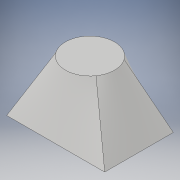
# Autodesk Inventor part: 410571040-4
Saved by Autodesk Inventor 2017 (Build 210142000, 142)
## iProperties
Part Number: 410571040-4
Material: 一般
Document SubType Name: Modeling
Designer: user
Density: 1 g/cm^3
Appearance: 預設
Author: user
Autodesk Inventor part; units mm, degrees
ref_plane "YZ Plane" through (0, 0, 0) normal (1, 0, 0) x (0, 1, 0)
ref_plane "XY Plane" through (0, 0, 0) normal (0, 0, 1) x (1, 0, 0)
sketch "草圖1" plane through (0, 0, 0) normal (0, 1, 0) x (-1, 0, 0)
  line L0 (0, 0) -> (-100, 0)
  line L1 (-100, 0) -> (-100, -70)
  line L2 (-100, -70) -> (0, -70)
  line L3 (0, -70) -> (0, 0)
  dimension "d0" = 100
  dimension "d1" = 70
  constraints: 8 end point, 3 perpendicular, 1 horizontal
  measures "d0" distance of L0.start L0.end
  measures "d1" distance of L2.end L0.start
ref_plane "工作平面1" through (0, 60, 0) normal (0, 1, 0) x (-1, 0, 0)
sketch "草圖2" plane through (0, 60, 0) normal (0, 1, 0) x (-1, 0, 0)
  circle A0 centre (-50, -35) radius 25
  point P0 (0, 0)
  dimension "d3" = 50
  dimension "d4" = 50
  dimension "d5" = 35
  constraints: 1 centre point
  measures "d3" diameter of A0
  measures "d4" horizontal distance of point (0, 0) A0.centre
  measures "d5" vertical distance of point (0, 0) A0.centre
loft "斷面混成1" add profiles "草圖1", "草圖2"
